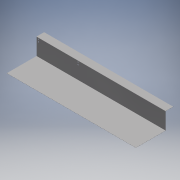
# Autodesk Inventor part: MC Part4
Saved by Autodesk Inventor 2016 (Build 200138000, 138)
## iProperties
Created: 2017-10-24
Part Number: MC Part4
Material: Steel, Mild
Document SubType Name: Sheet Metal
Designer: m207653
Density: 7.85 g/cm^3
Sheet Metal Rule: ms steel
Appearance: Semi-Polished
Flat Pattern Width: 67.9438 cm
Flat Pattern Length: 169.5 cm
Flat Pattern Area: 11516.5 cm^2
Sheet Metal Width: 679.438 mm
Sheet Metal Length: 1695.000 mm
Sheet Metal Area: 1151647.799 mm^2
Author: m207653
Autodesk Inventor part; units mm, degrees
ref_plane "YZ Plane" through (0, 0, 0) normal (1, 0, 0) x (0, 1, 0)
ref_plane "XZ Plane" through (0, 0, 0) normal (0, 1, 0) x (-1, 0, 0)
ref_plane "XY Plane" through (0, 0, 0) normal (0, 0, 1) x (1, 0, 0)
sketch "Sketch1" plane through (0, 0, 0) normal (0, 0, 1) x (1, 0, 0)
  line L0 (0, 0) -> (0, 392)
  line L1 (0, 392) -> (1695, 392)
  line L2 (1695, 392) -> (1695, 0)
  line L3 (1695, 0) -> (0, 0)
  dimension "d0" = 392
  dimension "d1" = 1695
  measures "d0" distance of L0.start L0.end
  measures "d1" distance of L0.end L1.end
extrude "Plate1" add sketch "Sketch1" along normal blind 1.6
sketch "Sketch2" plane through (1695, 390.4, 0) normal (0, 1, 0) x (-1, 0, 0)
  line L0 (1695, 0) -> (0, 0)
  line L1 (0, 0) -> (0, -223)
  line L2 (0, -223) -> (1695, -223)
  line L3 (1695, -223) -> (1695, 0)
  constraints: 6 end point, 1 horizontal, 1 perpendicular, 1 vertical
edge flange "Flange1" height 223 angle 90 thickness 1.6 bend radius 1.6 thickness toward (0, 1, 0) relief tear relief width 1.6 relief depth 0.8 edges at (847.5, 392, 0) wall of the first edge with corners at (0, 390.4, 0) (1695, 390.4, 0) (1695, 390.4, 223) (0, 390.4, 223)
bend "Bend1"
corner "Corner1"
sketch "Sketch3" plane through (0, 390.4, 221.4) normal (0, 0, 1) x (1, 0, 0)
  line L0 (1695, 0) -> (0, 0)
  line L1 (0, 0) -> (0, -70)
  line L2 (0, -70) -> (1695, -70)
  line L3 (1695, -70) -> (1695, 0)
  constraints: 6 end point, 1 horizontal, 1 perpendicular, 1 vertical
edge flange "Flange2" height 70 angle -90 thickness 1.6 bend radius 1.6 thickness toward (0, 0, 1) relief tear relief width 1.6 relief depth 0.8 edges at (847.5, 390.4, 223) wall of the first edge with corners at (1695, 390.4, 221.4) (0, 390.4, 221.4) (0, 460.4, 221.4) (1695, 460.4, 221.4)
bend "Bend2"
corner "Corner2"
sketch "Sketch4" plane through (0, 390.4, 3.2) normal (0, -1, 0) x (1, 0, 0)
  line L0 (0, 0) -> (0, 216.6) projected
  line L1 (0, 216.6) -> (0, 156.6)
  line L2 (0, 156.6) -> (1695, 156.6)
  line L3 (1695, 216.6) -> (1695, 0) projected
  line L4 (1695, 216.6) -> (0, 216.6) projected
  line L5 (1695, 156.6) -> (1695, 216.6)
  line L6 (1695, 216.6) -> (0, 216.6)
  circle A0 centre (25, 201.6) radius 6
  circle A1 centre (25, 171.6) radius 6
  circle A2 centre (545, 201.6) radius 6
  circle A3 centre (545, 171.6) radius 6
  line L7 (0, 156.6) -> (570, 156.6)
  line L8 (570, 156.6) -> (570, 216.6)
  point P0 (0, -3.2)
  dimension "d23" = 60
  dimension "d24" = 12
  dimension "d25" = 12
  dimension "d26" = 25
  dimension "d27" = 25
  dimension "d28" = 15
  dimension "d29" = 15
  dimension "d30" = 12
  dimension "d31" = 12
  dimension "d41" = 570
  dimension "d42" = 15
  dimension "d43" = 15
  dimension "d44" = 25
  dimension "d45" = 25
  constraints: 12 end point, 4 centre point, 4 point on line, 3 perpendicular, 1 vertical
  measures "d23" distance of L0.end L1.end
  measures "d24" diameter of A0
  measures "d25" diameter of A1
  measures "d26" distance from line of L0 A0.centre
  measures "d27" distance from line of L0 A1.centre
  measures "d28" distance from line of L4 A0.centre
  measures "d29" distance from line of L2 A1.centre
  measures "d30" diameter of A2
  measures "d31" diameter of A3
  measures "d41" distance of L1.end L7.end
  measures "d42" distance from line of L4 A2.centre
  measures "d43" distance from line of L2 A3.centre
  measures "d44" distance from line of L8 A2.centre
  measures "d45" distance from line of L8 A3.centre
hole "Hole1" at (25, 390.4, 204.8) at (25, 390.4, 174.8) at (545, 390.4, 204.8) at (545, 390.4, 174.8) direction (0, 1, 0) diameter 12 end through all
equation "\"d39\" = Thickness"
equation "\"d3\" = BendReliefWidth"
equation "\"d4\" = BendReliefDepth"
equation "\"d5\" = MinimumRemnant"
equation "\"d6\" = BendRadius"
equation "\"d9\" = BendRadius"
equation "\"d10\" = CornerReliefSize"
equation "\"d11\" = GapSize"
equation "\"d12\" = JacobiRadiusSize"
equation "\"d13\" = BendReliefWidth"
equation "\"d14\" = BendReliefDepth"
equation "\"d15\" = MinimumRemnant"
equation "\"d16\" = BendRadius"
equation "\"d19\" = BendRadius"
equation "\"d20\" = CornerReliefSize"
equation "\"d21\" = GapSize"
equation "\"d22\" = JacobiRadiusSize"
equation "\"BendRadius\" = Thickness"
equation "\"BendReliefWidth\" = Thickness"
equation "\"BendReliefDepth\" = 0.5 * Thickness"
equation "\"CornerReliefSize\" = 4 * Thickness"
equation "\"MinimumRemnant\" = 2 * Thickness"
equation "\"TransitionRadius\" = BendRadius"
equation "\"JacobiRadiusSize\" = BendRadius"
equation "\"GapSize\" = Thickness"
equation "\"d2\" = BendRadius"
equation "\"Thickness\" = 1.6"
body "Solid1"
